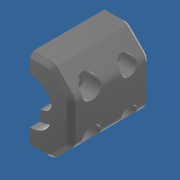
# Autodesk Inventor part: Print_Parts_N
Saved by Autodesk Inventor 2020 (Build 240168000, 168)
## iProperties
Created: 2020-10-05
Part Number: Print_Parts_N
Material: PC/ABS プラスチック
Document SubType Name: Modeling
Designer: kenta iguchi
Density: 0.357273 g/cm^3
Appearance: 滑らか - 黒
Author: kenta iguchi
Autodesk Inventor part; units mm, degrees
ref_plane "YZ Plane" through (0, 0, 0) normal (1, 0, 0) x (0, 1, 0)
ref_plane "XZ Plane" through (0, 0, 0) normal (0, 1, 0) x (-1, 0, 0)
ref_plane "XY Plane" through (0, 0, 0) normal (0, 0, 1) x (1, 0, 0)
sketch "スケッチ1" plane through (0, 0, 0) normal (0, 0, 1) x (1, 0, 0)
  circle A0 centre (0, 0) radius 20
  line L0 (0, 20) -> (0, -20)
  line L1 (-20, -20) -> (20, -20)
  line L2 (20, -20) -> (20, 20)
  line L3 (20, 20) -> (-20, 20)
  line L4 (-20, 20) -> (-20, -20)
  line L5 (-20, -20) -> (20, 20) construction
  line L6 (20, -20) -> (-20, 20) construction
  point P0 (20, 0)
  dimension "d0" = 40
  dimension "d9" = 40
  dimension "d10" = 40
  constraints: 14 end point, 2 midpoint, 2 parallel, 2 point on circle, 1 centre point, 1 coincident, 1 horizontal, 1 perpendicular, 1 vertical, 1 vertical alignment
  measures "d0" diameter of A0
  measures "d9" distance of L3.end L2.end
  measures "d10" distance of L2.end L1.end
extrude "押し出し1" add sketch "スケッチ1" along normal mid plane 20 contours A0 L0 | L2 L1 A0 | A0 L3 L2 picked at (5.2122, 4.1566)
sketch "スケッチ2" plane through (0, 0, 10) normal (0, 0, 1) x (1, 0, 0)
  line L0 (0, 20) -> (0, -20) projected
  circle A0 centre (0, 0) radius 11.1
  point P0 (0, 11.1)
  point P1 (0, -11.1)
  dimension "d3" = 22.2
  constraints: 1 centre point, 1 coincident
  measures "d3" diameter of A0
extrude "押し出し2" cut sketch "スケッチ2" against normal through all contours A0 L0 picked at (3.7161, 2.3997)
sketch "スケッチ3" plane through (0, 0, 0) normal (0, 0, 1) x (1, 0, 0)
  circle A0 centre (0, 0) radius 6
  arc A1 (0, -11.1) -> (0, 11.1) centre (0, 0) ccw projected
  line L0 (0, -11.1) -> (0, -20) projected
  line L1 (0, 20) -> (0, 11.1) projected
  line L2 (0, 11.1) -> (0, -11.1)
  line L3 (0, -20) -> (20, -20) projected
  line L4 (20, -20) -> (20, 20) projected
  line L5 (20, 20) -> (0, 20) projected
  point P0 (0, 6)
  point P1 (0, -6)
  dimension "d6" = 12
  constraints: 2 end point, 1 centre point, 1 coincident, 1 vertical
  measures "d6" diameter of A0
extrude "押し出し3" add sketch "スケッチ3" along normal mid plane 10 contours A0 L2 A1
chamfer "面取り1" distance 10 angle 45 2 edges at (20, 20, 0) (20, -20, 0)
sketch "スケッチ4" plane through (20, -10, -10) normal (1, 0, 0) x (0, 0, -1)
  line L0 (0, 30) -> (-20, 30) projected
  line L1 (-20, -10) -> (0, -10) projected
  point P0 (-10, 10)
  point P1 (-10, 20)
  point P2 (-10, 0)
  dimension "d14" = 10
  dimension "d15" = 10
  constraints: 2 vertical alignment
  measures "d14" distance from line of point (-10, 20) L0
  measures "d15" distance from line of point (-10, 0) L1
hole "穴1" at (20, 10, 0) at (20, -10, 0) direction (-1, 0, 0) diameter 5.3 depth 58 counterbore diameter 9.5 counterbore depth 8
sketch "Sketch5" plane through (0, 0, -10) normal (0, 0, -1) x (-1, 0, 0)
  line L0 (-10, -20) -> (-20, -10) projected
  line L1 (-10, -20) -> (0, -20) projected
  line L2 (0, -20) -> (0, -11.1) projected
  arc A0 (0, 11.1) -> (0, -11.1) centre (0, 0) ccw projected
  line L3 (0, 11.1) -> (0, 20) projected
  line L4 (0, 20) -> (-10, 20) projected
  line L5 (-20, 10) -> (-10, 20) projected
  line L6 (-20, 10) -> (-20, -10) projected
extrude "Extrusion4" add sketch "Sketch5" along normal blind 18
sketch "Sketch7" plane through (0, 0, -5) normal (0, 0, -1) x (-1, 0, 0)
  line L0 (0, -11.1) -> (0, -6) projected
  arc A0 (0, 6) -> (0, -6) centre (0, 0) ccw projected
  line L1 (0, 6) -> (0, 11.1) projected
  arc A1 (0, 11.1) -> (0, -11.1) centre (0, 0) ccw projected
extrude "Extrusion5" add sketch "Sketch7" along normal blind 18
sketch "Sketch6" plane through (20, -10, 10) normal (1, 0, 0) x (0, 0, -1)
  line L0 (14.75, 20) -> (38, 20) projected
  line L1 (38, 0) -> (14.75, 0) projected
  line L2 (0, 0) -> (0, 20) projected
  point P0 (10, 10)
  point P1 (28, 20)
  point P2 (28, 0)
  dimension "d25" = 28
  constraints: 2 point on line, 1 vertical alignment
  measures "d25" distance from line of point (28, 20) L2
hole "Hole2" at (20, 10, -18) at (20, -10, -18) direction (-1, 0, 0) diameter 4.3 depth 27.5 counterbore diameter 8 counterbore depth 8
fillet "Fillet1" radius 5 8 edges at (20, 10, 7.375) (20, 10, -9.375) (20, 10, -25) (20, -10, -25) (20, -10, -9.375) (20, -10, 7.375) (10, 20, -9) (10, -20, -9)
chamfer "Chamfer2" distance 2 angle 45 18 edges at (15, 15, 10) (19.6194, 9.8423, 10) (20, 0, 10) (19.6194, -9.8423, 10) (15, -15, 10) (9.8423, -19.6194, 10) (3.9645, -20, 10) (9.8423, 19.6194, 10) (3.9645, 20, 10) (15, 15, -28) (19.6194, 9.8423, -28) (20, 0, -28) (19.6194, -9.8423, -28) (15, -15, -28) (9.8423, -19.6194, -28) (3.9645, -20, -28) (9.8423, 19.6194, -28) (3.9645, 20, -28)
